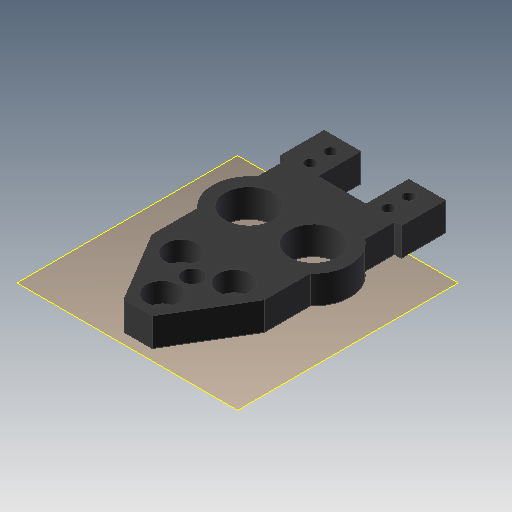
# Autodesk Inventor part: 30_Cube_Z_Focus_MGN_NEMA_slide_part2
Saved by Autodesk Inventor 2019.4 (Build 234330000, 330)
## iProperties
Created: 2021-04-25
Part Number: 30_Cube_Z_Focus_MGN_NEMA_slide_part2
Material: Generic
Document SubType Name: Modeling
Designer: diederichbenedict
Density: 1 g/cm^3
Appearance: Default
Author: diederichbenedict
Autodesk Inventor part; units mm, degrees
ref_plane "YZ Plane" through (0, 0, 0) normal (1, 0, 0) x (0, 1, 0)
ref_plane "XZ Plane" through (0, 0, 0) normal (0, 1, 0) x (-1, 0, 0)
ref_plane "XY Plane" through (0, 0, 0) normal (0, 0, 1) x (1, 0, 0)
ref_plane "Work Plane8" through (-7.4556, -16.4352, 24.63) normal (0, 1, 0) x (0, 0, -1)
sketch "Sketch12" plane through (-7.4556, -16.4352, 24.63) normal (0, 1, 0) x (0, 0, -1)
  circle A0 centre (31.71, -8) radius 6 construction
  circle A1 centre (31.71, 8) radius 6 construction
  line L0 (59.1648, 4.9103) -> (72.1552, 12.4103) construction
  arc A2 (80.66, 7.5) -> (72.1552, 12.4103) centre (70.66, 0) ccw construction
  line L1 (80.66, 7.5) -> (80.66, -7.5) construction
  arc A3 (72.1552, -12.4103) -> (80.66, -7.5) centre (70.66, 0) ccw construction
  line L2 (72.1552, -12.4103) -> (59.1648, -4.9103) construction
  arc A4 (59.1648, 4.9103) -> (59.1648, -4.9103) centre (70.66, 0) ccw construction
  line L3 (57.3131, 5.945) -> (46.6951, 5.945) construction
  line L4 (46.6951, 5.945) -> (46.6951, -5.9961)
  line L5 (46.6951, -5.9961) -> (57.3131, -5.9961)
  line L6 (57.3131, -5.9961) -> (57.3131, -15)
  line L7 (57.3131, -15) -> (85.66, -15) construction
  line L8 (85.66, -15) -> (85.66, 15) construction
  line L9 (85.66, 15) -> (57.3131, 15) construction
  line L10 (57.3131, 15) -> (57.3131, 5.945) construction
  line L11 (46.6951, -6.3061) -> (57.3131, -6.3061)
  line L12 (3.89, -16.97) -> (37.83, -16.97)
  line L13 (41.63, -16.87) -> (45.71, -16.87)
  line L14 (55.66, -15) -> (46.2855, -13.3689)
  line L15 (55.66, -15) -> (105.1976, -15) construction
  line L16 (46.6951, 0) -> (46.6951, -6.3061)
  arc A5 (24.9318, -13.9208) -> (37.3669, -15) centre (31.71, -8) ccw
  line L17 (24.9318, -13.9208) -> (13.5861, -13.9208)
  line L18 (-3.79, -3.4952) -> (-3.79, 3.4952)
  line L19 (-3.79, 0) -> (-3.79, 0)
  line L20 (-3.79, 0) -> (-3.79, -3.4952)
  line L21 (-3.79, -3.4952) -> (13.5861, -13.9208)
  line L22 (46.6951, 0) -> (-3.79, 0)
  line L23 (57.3131, -6.3061) -> (57.3131, -15)
  line L24 (57.3131, -15) -> (37.3669, -15)
  line L25 (-3.79, -8.16) -> (-3.79, 8.16)
  line L26 (19.46, 16.4952) -> (10.1021, 16.4952)
  line L27 (19.46, -16.4952) -> (19.46, 16.4952)
  line L28 (10.1021, -16.4952) -> (19.46, -16.4952)
  line L29 (10.1021, 16.4952) -> (-3.79, 8.16)
  line L30 (-3.79, -8.16) -> (10.1021, -16.4952)
  circle A6 centre (9.71, 0) radius 1.75
  point P0 (24.63, -7.4556)
  point P1 (11.21, -12.4952)
  point P2 (19.46, 12.4952)
  point P3 (19.46, -12.4952)
extrude "Extrusion11" add sketch "Sketch12" along normal blind 7 contours L4 L16 L11 L6 L24 A5 L12 L17 L27 L22 | L5 L6 L11 L16 | L27 L17 L21 L18 L22 A6 | A6 L22 | L12 A5 picked at (9.6397, -0.5791)
sketch "Sketch13" plane through (-7.4556, -9.4352, 24.63) normal (0, 1, 0) x (1, 0, 0)
  circle A0 centre (8, 31.71) radius 6 projected
  circle A1 centre (8, 31.71) radius 6.1
  circle A2 centre (9.6825, 53.6267) radius 1.4 projected
  circle A3 centre (9.6825, 48.6267) radius 1.4 projected
  circle A4 centre (0, 9.71) radius 2.5 projected
  point P0 (7.4556, 24.63)
  dimension "d68" = 12.2
  constraints: 1 centre point, 1 coincident
  measures "d68" diameter of A1
extrude "Extrusion12" cut sketch "Sketch13" against normal through all contours A0 | A2 | A3 | A4
sketch "Sketch16" plane through (-7.4556, -9.4352, 24.63) normal (0, 1, 0) x (1, 0, 0)
  line L0 (13.9208, 13.5861) -> (13.9208, 24.9318) projected
  arc A0 (13.9208, 24.9318) -> (15, 37.3669) centre (8, 31.71) ccw projected
  line L1 (5.9961, 46.6951) -> (0, 46.6951) projected
  line L2 (13.8689, 40.3869) -> (13.8689, 45.71) projected
  line L3 (15, 39.0186) -> (13.3086, 39.0186)
  line L4 (13.3086, 39.0186) -> (13.3086, 46.45)
  line L5 (13.3086, 46.45) -> (15, 46.45)
  line L6 (15, 46.45) -> (15, 39.0186)
  arc A1 (15, 37.3669) -> (13.3086, 39.0186) centre (7.8235, 31.71) ccw
  line L7 (13.3086, 46.45) -> (15, 48.1414)
  line L8 (15, 37.3669) -> (15, 57.3131) projected
  line L9 (13.3086, 46.45) -> (15.7006, 46.45) construction
  line L10 (15, 48.1414) -> (15, 46.45)
  line L11 (15, 39.0186) -> (15, 37.3669)
  line L12 (0, 7.21) -> (0, -3.79) projected
  line L13 (0, -3.79) -> (3.4952, -3.79) projected
  line L14 (3.4952, -3.79) -> (13.9208, 13.5861) projected
  line L15 (15, 37.3669) -> (15, 57.3131) projected
  line L16 (15, 57.3131) -> (5.9961, 57.3131) projected
  line L17 (5.9961, 57.3131) -> (5.9961, 46.6951) projected
  arc A2 (0, 7.21) -> (0, 12.21) centre (0, 9.71) ccw projected
  line L18 (0, 46.6951) -> (0, 12.21) projected
  point P0 (7.4556, 24.63)
  dimension "d80" = 45
  constraints: 16 end point, 4 point on line, 2 horizontal, 2 parallel, 2 point on circle, 1 centre point, 1 equal length, 1 perpendicular, 1 vertical
  measures "d80" angle of L9 L7
extrude "Extrusion15" cut sketch "Sketch16" against normal through all contours A1 L3 L8 | L4 L5 L6 L3
mirror "Mirror3" about plane through (-7.4556, -16.4352, -22.0651) normal (-1, 0, 0) of "Extrusion11", "Extrusion12", "Extrusion15"
sketch "Sketch17" plane through (-7.4556, -9.4352, 24.63) normal (0, 1, 0) x (1, 0, 0)
  circle A0 centre (6.4952, 13.46) radius 4 projected
  circle A1 centre (0, 2.21) radius 4 projected
  circle A2 centre (-6.4952, 13.46) radius 4 projected
  point P0 (7.4556, 24.63)
extrude "Extrusion16" cut sketch "Sketch17" against normal blind 5
body "Solid2"
